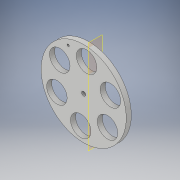
# Autodesk Inventor part: threaded filter wheel
Saved by Autodesk Inventor 2017 (Build 210142000, 142)
## iProperties
Created: 2016-09-01
Part Number: threaded filter wheel
Material: Generic
Document SubType Name: Modeling
Designer: Darien Morrow
Density: 1 g/cm^3
Appearance: Default
Author: Darien Morrow
Autodesk Inventor part; units mm, degrees
ref_plane "XZ Plane" through (0, 0, 0) normal (0, 1, 0) x (-1, 0, 0)
ref_plane "XY Plane" through (0, 0, 0) normal (0, 0, 1) x (1, 0, 0)
sketch "Sketch1" plane through (0, 0, 0) normal (0, 0, 1) x (1, 0, 0)
  circle A0 centre (0, 0) radius 53.34
  dimension "d0" = 106.68
  constraints: 1 centre point, 1 coincident
  measures "d0" diameter of A0
extrude "Extrusion1" add sketch "Sketch1" along normal mid plane 6.35
sketch "Sketch2" plane through (0, 0, -3.175) normal (0, 0, -1) x (-1, 0, 0)
  point P0 (0, 0)
sketch "Sketch3" plane through (0, 0, -3.175) normal (0, 0, -1) x (-1, 0, 0)
  line L0 (29.9214, 21.4747) -> (33.5583, -15.1753)
  line L1 (33.5583, -15.1753) -> (3.6369, -36.65)
  line L2 (3.6369, -36.65) -> (-29.9214, -21.4747)
  line L3 (-29.9214, -21.4747) -> (-33.5583, 15.1753)
  line L4 (-33.5583, 15.1753) -> (-3.6369, 36.65)
  line L5 (-3.6369, 36.65) -> (29.9214, 21.4747)
  point P0 (0, 0)
  point P1 (0, 0)
  dimension "d3" = 36.83
  constraints: 12 end point, 7 coincident, 13 other
  measures "d3" distance of L0.start point (0, 0)
hole "Hole1" at (33.5583, 15.1753, -3.175) at (3.6369, 36.65, -3.175) at (-29.9214, 21.4747, -3.175) at (-33.5583, -15.1753, -3.175) at (-3.6369, -36.65, -3.175) at (29.9214, -21.4747, -3.175) direction (0, 0, 1) diameter 25.6794 end through all
sketch "Sketch4" plane through (0, 0, -3.175) normal (0, 0, -1) x (-1, 0, 0)
  circle A0 centre (0, 0) radius 6.35
  dimension "d11" = 12.7
  constraints: 1 centre point, 1 coincident
  measures "d11" diameter of A0
extrude "Extrusion2" add sketch "Sketch4" along normal blind 9.525
sketch "Sketch5" plane through (0, 0, -12.7) normal (0, 0, -1) x (-1, 0, 0)
  circle A0 centre (0, 0) radius 6.35 projected
  constraints: 1 coincident
hole "Hole2" at (0, 0, -12.7) direction (0, 0, 1) diameter 5.08 end through all
ref_plane "Work Plane1" through (6.35, 0, 0) normal (1, 0, 0) x (0, 1, 0)
sketch "Sketch6" plane through (6.35, 0, 0) normal (1, 0, 0) x (0, 1, 0)
  line L0 (-6.35, -12.7) -> (6.35, -12.7) projected
  point P0 (0, 0)
  point P1 (0, -9.525)
  dimension "d22" = 3.175
  measures "d22" distance from line of point (0, -9.525) L0
hole "Hole3" at (6.35, 0, -9.525) direction (-1, 0, 0) diameter 2.159 depth 6.35 tip angle 118
sketch "Sketch7" plane through (0, 0, 3.175) normal (0, 0, 1) x (1, 0, 0)
  circle A0 centre (0, 0) radius 2.54 projected
  line L0 (0, 0) -> (-21.9781, 48.6017)
  circle A1 centre (0, 0) radius 53.34 projected
  circle A2 centre (-29.9214, 21.4747) radius 12.8397 projected
  line L1 (-29.9214, 21.4747) -> (3.4827, 36.5803)
  line L2 (3.4827, 36.5803) -> (3.4827, 23.8112)
  circle A3 centre (3.6369, 36.65) radius 12.8397 projected
  line L3 (3.4827, 36.5803) -> (-8.5593, 40.6638)
  line L4 (-21.9781, 48.6017) -> (-19.3657, 42.8249)
  dimension "d30" = 12.7155
  dimension "d31" = 5.5753
  constraints: 10 end point, 2 point on circle, 1 coincident, 1 perpendicular, 1 point on line, 1 vertical, 2 other
  measures "d30" distance of L1.end L3.end
  measures "d31" distance edge to line of A3 L0
hole "Hole4" at (-19.3657, 42.8249, 3.175) direction (0, 0, -1) diameter 2.6416 end through all thread size "6-32 UNC" class "2B" standard "ANSI Unified Screw Threads"
body "Solid1"
